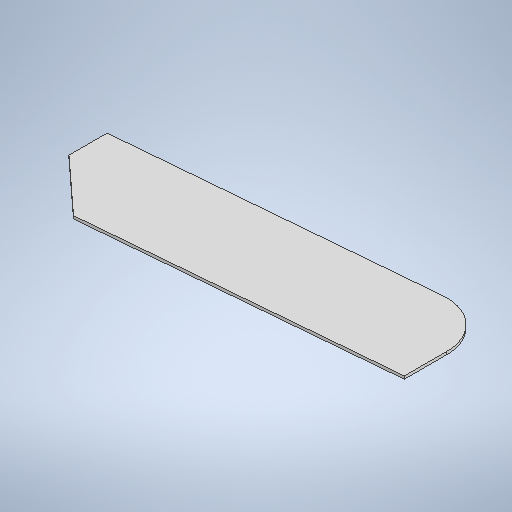
# Autodesk Inventor part: b
Saved by Autodesk Inventor 2025.2 (Build 292293000, 293)
## iProperties
Created: 2026-02-05
Part Number: b
Material: Generic
Document SubType Name: Modeling
Designer: Joefi
Density: 1 g/cm^3
Appearance: Default
Author: Joefi
Autodesk Inventor part; units mm, degrees
ref_plane "YZ Plane" through (0, 0, 0) normal (1, 0, 0) x (0, 1, 0)
ref_plane "XZ Plane" through (0, 0, 0) normal (0, 1, 0) x (-1, 0, 0)
ref_plane "XY Plane" through (0, 0, 0) normal (0, 0, 1) x (1, 0, 0)
sketch "Sketch1" plane through (0, 0, 0) normal (0, 1, 0) x (-1, 0, 0)
  line L0 (49.2661, -2.3961) -> (33.9381, 11.6495)
  line L1 (33.9381, 11.6495) -> (-51.3533, 4.1874)
  line L2 (-51.3533, 4.1874) -> (-51.3533, -7.7249)
  arc A0 (-51.3533, -7.7249) -> (-37.2203, -20.6754) centre (-38.3533, -7.7249) ccw
  line L3 (-37.2203, -20.6754) -> (49.2661, -13.1088)
  line L4 (49.2661, -13.1088) -> (49.2661, -2.3961)
  arc A1 (-49.3533, -7.7249) -> (-37.3946, -18.683) centre (-38.3533, -7.7249) ccw
  line L5 (-49.3533, -7.7249) -> (-49.3533, -2.2269)
  arc A2 (-44.7891, 2.7541) -> (-49.3533, -2.2269) centre (-44.3533, -2.2269) ccw
  line L6 (-44.7891, 2.7541) -> (31.044, 9.3886)
  arc A3 (34.8577, 8.094) -> (31.044, 9.3886) centre (31.4798, 4.4077) ccw
  line L7 (34.8577, 8.094) -> (45.6441, -1.7898)
  arc A4 (47.2661, -5.4762) -> (45.6441, -1.7898) centre (42.2661, -5.4762) ccw
  line L8 (47.2661, -5.4762) -> (47.2661, -6.6945)
  arc A5 (42.7019, -11.6755) -> (47.2661, -6.6945) centre (42.2661, -6.6945) ccw
  line L9 (42.7019, -11.6755) -> (-37.3946, -18.683)
  line L10 (-51.1533, 4.0042) -> (33.8678, 11.4426)
  line L11 (33.8678, 11.4426) -> (49.0661, -2.4841)
  line L12 (49.0661, -2.4841) -> (49.0661, -12.9256)
  line L13 (49.0661, -12.9256) -> (-37.2377, -20.4762)
  arc A6 (-51.1533, -7.7249) -> (-37.2377, -20.4762) centre (-38.3533, -7.7249) ccw
  line L14 (-51.1533, -7.7249) -> (-51.1533, 4.0042)
  point P0 (0, 0)
  dimension "d0" = 0.2
  constraints: 30 end point, 14 point on circle, 7 centre point, 5 other
  measures "d0" distance between parallel lines of L1 L10
extrude "Extrusion1" add sketch "Sketch1" along normal blind 0.8 contours L4 L3 A0 L2 L1 L0 | L5 A2 L6 A3 L7 A4 L8 A5 L9 A1 | L10 L11 L12 L13 A6 L14
body "Solid1"
